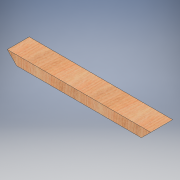
# Autodesk Inventor part: 22_9 Inch 45 Diagonal Piece
Saved by Autodesk Inventor 2016 (Build 200138000, 138)
## iProperties
Created: 2015-07-05
Part Number: 22_9 Inch 45 Diagonal Piece
Material: Wood (Birch)
Document SubType Name: Modeling
Designer: steele
Density: 0.55 g/cm^3
Appearance: Birch - Natural Polished
Author: steele
Autodesk Inventor part; units mm, degrees
ref_plane "YZ Plane" through (0, 0, 0) normal (1, 0, 0) x (0, 1, 0)
ref_plane "XZ Plane" through (0, 0, 0) normal (0, 1, 0) x (-1, 0, 0)
ref_plane "XY Plane" through (0, 0, 0) normal (0, 0, 1) x (1, 0, 0)
sketch "Sketch2" plane through (0, 0, 0) normal (0, 0, 1) x (1, 0, 0)
  line L0 (-262.0465, -22.8928) -> (243.4135, -22.8928)
  line L1 (281.5135, 15.2072) -> (-300.1465, 15.2072)
  line L2 (-299.4939, -16.1784) -> (281.5135, 15.2072) construction
  line L3 (280.9626, -14.2352) -> (-300.1465, 15.2072) construction
  line L4 (-300.1465, 15.2072) -> (-262.0465, -22.8928)
  line L5 (-300.1465, 15.2072) -> (-246.2649, 15.2072) construction
  line L6 (281.5135, 15.2072) -> (243.4135, -22.8928)
  line L7 (281.5135, 15.2072) -> (335.3951, 15.2072) construction
  point P0 (0, 0)
  dimension "d10" = 45
  dimension "d11" = 135
  dimension "d14" = 581.66
  dimension "d15" = 38.1
  constraints: 16 end point, 3 horizontal, 2 equal length, 2 point on line, 1 parallel
  measures "d10" angle of L4 L5
  measures "d11" angle of L6 L7
  measures "d14" distance of L1.start L1.end
  measures "d15" distance between parallel lines of L0 L1
extrude "Extrusion2" add sketch "Sketch2" along normal mid plane 88.9
body "Solid2"
